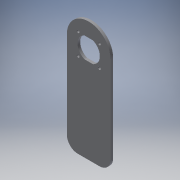
# Autodesk Inventor part: pG188Mount
Saved by Autodesk Inventor 2018 (Build 220112000, 112)
## iProperties
Created: 2017-02-20
Part Number: pG188Mount
Material: Generic
Document SubType Name: Sheet Metal
Designer: kingb
Density: 1 g/cm^3
Sheet Metal Rule: Default
Appearance: Default
Author: kingb
Autodesk Inventor part; units mm, degrees
ref_plane "YZ Plane" through (0, 0, 0) normal (1, 0, 0) x (0, 1, 0)
ref_plane "XZ Plane" through (0, 0, 0) normal (0, 1, 0) x (-1, 0, 0)
ref_plane "XY Plane" through (0, 0, 0) normal (0, 0, 1) x (1, 0, 0)
sketch "Sketch1" plane through (0, 0, 0) normal (0, 0, 1) x (1, 0, 0)
  line L0 (0, 0) -> (50.8, 0)
  line L1 (50.8, 0) -> (50.8, 27.1979)
  line L2 (50.8, 139.7) -> (0, 139.7) construction
  line L3 (0, 139.7) -> (0, 0)
  line L4 (128.6063, 161.9886) -> (104.1161, 68.3618)
  line L5 (418.4795, 73.9788) -> (-1.9313, 310.0684)
  arc A0 (104.1161, 68.3618) -> (50.8, 27.1979) centre (93.3487, 27.1979) ccw construction
  line L6 (128.6063, 161.9886) -> (145.6601, 227.1856)
  line L7 (63.1831, 62.4318) -> (91.6427, 171.2335) construction
  arc A1 (50.8, 139.7) -> (91.6427, 171.2335) centre (50.8, 181.9168) ccw
  line L8 (95.8188, 187.1988) -> (111.3222, 246.4687)
  line L9 (91.6427, 171.2335) -> (95.8188, 187.1988)
  line L10 (50.8, 27.1979) -> (50.8, 139.7)
  line L11 (417.0097, 172.2938) -> (-48.9451, 294.1693)
  line L12 (50.8, 139.7) -> (50.8, 268.0799)
  line L13 (50.8, 268.0799) -> (0, 268.0799)
  line L14 (0, 268.0799) -> (0, 139.7)
  dimension "d0" = 50.8
  dimension "d1" = 139.7
  measures "d0" distance of L2.end L2.start
  measures "d1" distance of L2.start L0.end
extrude "Plate1" add sketch "Sketch1" along normal blind 3.048 contours L3 L14 L13 L12 L10 L1 L0
fillet "Corner Round2" radius 12.7 2 edges at (50.8, 0, 1.524) (0, 0, 1.524)
sketch "Sketch2" plane through (0, 0, 0) normal (0, 0, -1) x (-1, 0, 0)
  arc A0 (-20.4, 99.125) -> (-20.4, 123.125) centre (-25.4, 111.125) ccw projected
  line L0 (-20.4, 123.125) -> (-30.4, 123.125) projected
  line L1 (-30.4, 99.125) -> (-20.4, 99.125) projected
  arc A1 (-30.4, 123.125) -> (-30.4, 99.125) centre (-25.4, 111.125) ccw projected
  circle A2 centre (-13.0256, 98.7506) radius 1.65 projected
  circle A3 centre (-37.7744, 123.4994) radius 1.65 projected
  circle A4 centre (-13.0256, 123.4994) radius 1.65 projected
  circle A5 centre (-37.7744, 98.7506) radius 1.65 projected
  point P0 (0, 0)
extrude "Extrusion1" cut sketch "Sketch2" against normal up to surface (3.048 mm away)
fillet "Corner Round4" radius 25.4 2 edges at (50.8, 268.0799, 1.524) (0, 268.0799, 1.524)
sketch "Sketch6" plane through (0, 0, 3.048) normal (0, 0, 1) x (1, 0, 0)
  line L0 (406.4, 135.7009) -> (-31.623, 262.7009) construction
  circle A0 centre (25.4, 246.1677) radius 3.175
  arc A1 (50.8, 242.6799) -> (0, 242.6799) centre (25.4, 242.6799) ccw projected
  point P0 (0, 0)
  dimension "d33" = 6.35
  dimension "d34" = 0
  constraints: 1 centre point, 1 point on line
  measures "d33" diameter of A0
  measures "d34" horizontal distance of A1.centre A0.centre
extrude "Extrusion4" cut sketch "Sketch6" against normal up to next
sketch "Sketch7" plane through (0, 0, 3.048) normal (0, 0, 1) x (1, 0, 0)
  circle A0 centre (12.7, 19.05) radius 3.175
  circle A1 centre (38.1, 19.05) radius 3.175
  line L0 (38.1, 0) -> (12.7, 0) projected
  line L1 (0, 12.7) -> (0, 242.6799) projected
  line L2 (50.8, 242.6799) -> (50.8, 12.7) projected
  point P0 (0, 0)
  dimension "d37" = 6.35
  dimension "d38" = 6.35
  dimension "d39" = 19.05
  dimension "d40" = 12.7
  dimension "d41" = 12.7
  constraints: 2 centre point, 1 horizontal alignment
  measures "d37" diameter of A0
  measures "d38" diameter of A1
  measures "d39" distance from line of L0 A0.centre
  measures "d40" distance from line of L1 A0.centre
  measures "d41" distance from line of L2 A1.centre
extrude "Extrusion5" cut sketch "Sketch7" against normal up to next
equation "\"d10\" = Thickness"
equation "\"BendRadius\" = Thickness"
equation "\"BendReliefWidth\" = Thickness"
equation "\"BendReliefDepth\" = 0.5 * Thickness"
equation "\"CornerReliefSize\" = 4 * Thickness"
equation "\"MinimumRemnant\" = 2 * Thickness"
equation "\"TransitionRadius\" = BendRadius"
equation "\"JacobiRadiusSize\" = Thickness"
equation "\"GapSize\" = Thickness"
equation "\"d2\" = BendRadius"
equation "\"Thickness\" = 3.048"
body "Solid1"
